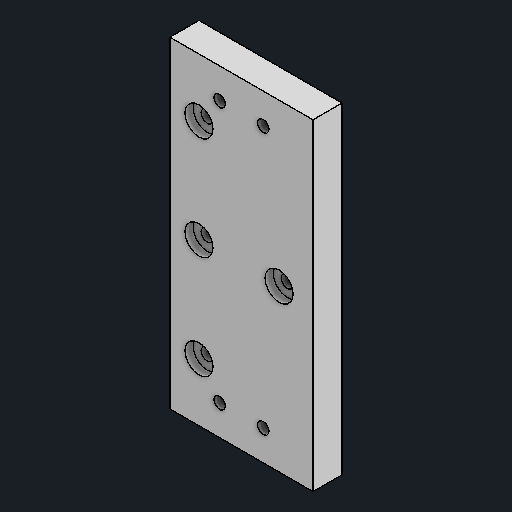
# Autodesk Inventor part: Fixed Side Adapter Plate
Saved by Autodesk Inventor 2026.2 (Build 302298000, 298)
## iProperties
Created: 2026-04-18
Part Number: Fixed Side Adapter Plate
Material: Generic
Document SubType Name: Modeling
Designer: JoshuaEah
Density: 1 g/cm^3
Appearance: Default
Author: JoshuaEah
Autodesk Inventor part; units mm, degrees
ref_plane "YZ Plane" through (0, 0, 0) normal (1, 0, 0) x (0, 1, 0)
ref_plane "XZ Plane" through (0, 0, 0) normal (0, 1, 0) x (-1, 0, 0)
ref_plane "XY Plane" through (0, 0, 0) normal (0, 0, 1) x (1, 0, 0)
sketch "Sketch1" plane through (0, 0, 0) normal (0, 0, 1) x (1, 0, 0)
  line L0 (0, 0) -> (62.5348, 0)
  line L1 (62.5348, 0) -> (62.5348, 140.716)
  line L2 (62.5348, 140.716) -> (0, 140.716)
  line L3 (0, 140.716) -> (0, 0)
  line L4 (0, 70.358) -> (62.5348, 70.358)
  circle A0 centre (12.7, 70.358) radius 2.5
  circle A1 centre (12.7, 115.358) radius 2.5
  circle A2 centre (12.7, 25.358) radius 2.5
  circle A3 centre (21.7424, 127.508) radius 3.175
  circle A4 centre (21.7424, 13.208) radius 3.175
  circle A5 centre (40.7924, 127.508) radius 3.175
  circle A6 centre (40.7924, 13.208) radius 3.175
  circle A7 centre (47.7, 70.358) radius 2.5
  dimension "d0" = 140.716
  dimension "d1" = 5
  dimension "d2" = 12.7
  dimension "d3" = 45
  dimension "d5" = 6.35
  dimension "d6" = 114.3
  dimension "d10" = 19.05
  dimension "d16" = 35
  dimension "d33" = 62.5348
  dimension "d34" = 21.7424
  dimension "d35" = 21.7424
  constraints: 10 end point, 8 centre point, 2 equal radius, 2 horizontal, 2 midpoint, 2 parallel, 2 point on line, 2 symmetric about line, 1 perpendicular, 1 vertical alignment, 6 other
  measures "d0" distance of L0.end L1.end
  measures "d1" diameter of A0
  measures "d2" distance from line of L3 A0.centre
  measures "d3" distance of A0.centre A1.centre
  measures "d5" diameter of A3
  measures "d6" diameter of A3.centre L4
  measures "d10" distance of A3.centre A5.centre
  measures "d16" distance of A0.centre A7.centre
  measures "d33" distance of L1.end L2.end
  measures "d34" distance from line of L3 A3.centre
  measures "d35" distance from line of L1 A5.centre
extrude "Extrusion1" add sketch "Sketch1" against normal blind 12.7 contours L3 L4 A0 A7 L1 L0 | L3 L2 L1 L4 A7 A0 | A0 L4 | L4 A0 | A7 L4 | L4 A7 | A1 | A2 | A3 | A4 | A5 | A6
hole "Hole1" at (12.7, 115.358, 0) at (12.7, 70.358, 0) at (12.7, 25.358, 0) at (47.7, 70.358, 0) direction (0, 0, -1) diameter 5.3086 end through all counterbore diameter 12.2428 counterbore depth 3.5814 clearance for "Hex Head Bolt" size "M5" standard "Ansi Metric M Profile"
hole "Hole2" at (21.7424, 13.208, 0) at (40.7924, 13.208, 0) at (40.7924, 127.508, 0) at (21.7424, 127.508, 0) direction (0, 0, -1) diameter 4.9784 end through all thread size "1/4-20 UNC" class "2B" standard "ANSI Unified Screw Threads"
equation "\"d34\" = d35"
body "Solid1"
